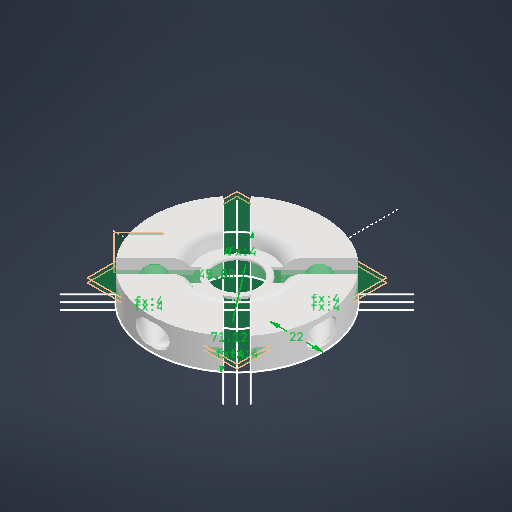
# Autodesk Inventor part: CENTER RING
Saved by Autodesk Inventor 2025 (Build 290162010, 162A)
## iProperties
Created: 2025-07-06
Part Number: CENTER RING
Material: Generic
Document SubType Name: Modeling
Designer: Jebediah Kerman
Density: 1 g/cm^3
Appearance: Default
Author: Jebediah Kerman
Autodesk Inventor part; units mm, degrees
ref_plane "YZ Plane" through (0, 0, 0) normal (1, 0, 0) x (0, 1, 0)
ref_plane "XZ Plane" through (0, 0, 0) normal (0, 1, 0) x (-1, 0, 0)
ref_plane "XY Plane" through (0, 0, 0) normal (0, 0, 1) x (1, 0, 0)
sketch "Sketch1" plane through (0, 0, 0) normal (0, 1, 0) x (-1, 0, 0)
  circle A0 centre (0, 0) radius 35.56
  circle A1 centre (0, 0) radius 13.56
  line L0 (0, 0) -> (36.4898, -36.4898)
  line L1 (0, 0) -> (51.6043, 0) construction
  line L2 (0, 0) -> (0, -67.3303) construction
  line L3 (0, 0) -> (-36.4898, -36.4898)
  line L4 (0, 0) -> (36.4898, 36.4898)
  line L5 (0, 0) -> (-36.4898, 36.4898)
  line L6 (-2.8284, 2.8284) -> (-39.3182, -33.6614)
  line L7 (2.8284, -2.8284) -> (-33.6614, -39.3182)
  line L8 (-2.8284, -2.8284) -> (-39.3182, 33.6614)
  line L9 (2.8284, 2.8284) -> (-33.6614, 39.3182)
  line L10 (2.8284, -2.8284) -> (39.3182, 33.6614)
  line L11 (-2.8284, 2.8284) -> (33.6614, 39.3182)
  line L12 (2.8284, 2.8284) -> (39.3182, -33.6614)
  line L13 (-2.8284, -2.8284) -> (33.6614, -39.3182)
  point P0 (11.9901, 6.3333)
  point P1 (27.8136, 22.1567)
  point P2 (22.1567, 27.8136)
  point P3 (6.3333, 11.9901)
  point P4 (6.3333, -11.9901)
  point P5 (22.1567, -27.8136)
  point P6 (27.8136, -22.1567)
  point P7 (11.9901, -6.3333)
  point P8 (-11.9901, -6.3333)
  point P9 (-27.8136, -22.1567)
  point P10 (-22.1567, -27.8136)
  point P11 (-6.3333, -11.9901)
  point P12 (-27.8136, 22.1567)
  point P13 (-11.9901, 6.3333)
  point P14 (-6.3333, 11.9901)
  point P15 (-22.1567, 27.8136)
  dimension "d0" = 71.12
  dimension "d1" = 22
  dimension "d4" = 45
  dimension "d5" = 4
  dimension "d6" = 4
  dimension "d7" = 4
  dimension "d8" = 4
  dimension "d9" = 4
  dimension "d10" = 4
  dimension "d11" = 4
  dimension "d12" = 4
  constraints: 28 end point, 8 parallel, 3 symmetric about line, 2 centre point, 1 coincident, 1 equal length, 1 horizontal, 1 vertical
  measures "d0" diameter of A0
  measures "d1" radial gap between concentric circles of A0 A1
  measures "d4" angle of L0 L1
  measures "d5" distance between parallel lines of L3 L6
  measures "d6" distance between parallel lines of L3 L7
  measures "d7" distance between parallel lines of L5 L8
  measures "d8" distance between parallel lines of L5 L9
  measures "d9" distance between parallel lines of L4 L10
  measures "d10" distance between parallel lines of L4 L11
  measures "d11" distance between parallel lines of L0 L12
  measures "d12" distance between parallel lines of L0 L13
extrude "Extrusion1" add sketch "Sketch1" along normal blind 13 contours A0 L12 A1 L10 | L10 A1 L4 A0 | A0 L0 A1 L12 | L4 A1 L11 A0 | A0 L13 A1 L0 | L11 A1 L9 A0 | A0 L7 A1 L13 | L9 A1 L5 A0 | A0 L3 A1 L7 | L5 A1 L8 A0 | A0 L6 A1 L3 | L8 A1 L6 A0
extrude "Extrusion2" cut sketch "Sketch1" along normal blind 13 contours L10 A1 L4 A0 | A0 L0 A1 L12 | L4 A1 L11 A0 | A0 L13 A1 L0 | L9 A1 L5 A0 | A0 L3 A1 L7 | L5 A1 L8 A0 | A0 L6 A1 L3
ref_plane "Work Plane1" through (-36.2988, 0, 13.6714) normal (-0.7071068, 0, -0.7071068) x (-0.7071068, 0, 0.7071068)
sketch "Sketch2" plane through (-36.2988, 0, 13.6714) normal (-0.7071068, 0, -0.7071068) x (-0.7071068, 0, 0.7071068)
  line L0 (0, 0) -> (-31.3343, 0) projected
  line L1 (-22.3777, 13) -> (-22.3777, 0) projected
  line L2 (0, 0) -> (-22.3777, 13) construction
  line L3 (0, 0) -> (0, 13) projected
  line L4 (-22.3777, 0) -> (0, 13) construction
  circle A0 centre (-11.1889, 6.5) radius 4.5
  point P0 (-35.3343, 0)
  dimension "d16" = 9
  constraints: 4 end point, 1 centre point, 1 coincident, 1 midpoint
  measures "d16" diameter of A0
extrude "Extrusion3" cut sketch "Sketch2" along normal blind 13 and the other way blind 50
mirror "Mirror1" about plane through (0, 0, 0) normal (1, 0, 0) of "Extrusion3"
mirror "Mirror2" about plane through (0, 0, 0) normal (0, 0, 1) of "Extrusion3", "Mirror1"
fillet "Fillet1" radius 6 4 edges at (13.56, 13, 0) (0, 13, 13.56) (-13.56, 13, 0) (0, 13, -13.56)
ref_plane "Work Plane3" through (0, 8.75, 0) normal (0, -1, 0) x (1, 0, 0)
ref_plane "Work Plane2" through (0, 7, 0) normal (0, -1, 0) x (1, 0, 0)
sketch "Sketch4" plane through (0, 8.75, 0) normal (0, -1, 0) x (1, 0, 0)
  circle A0 centre (0, 0) radius 11
  line L0 (27.8136, 22.1567) -> (11.9901, 6.3333) projected
  circle A1 centre (0, 0) radius 14.2522
  line L1 (11.9901, -6.3333) -> (27.8136, -22.1567) projected
  line L2 (12.5012, -6.8444) -> (-6.8444, 12.5012)
  line L3 (-12.5012, 6.8444) -> (6.8444, -12.5012)
  line L4 (-6.8444, -12.5012) -> (12.5012, 6.8444)
  line L5 (6.8468, 12.4999) -> (-12.4999, -6.8468)
  circle A2 centre (0, 0) radius 8.5
  point P0 (6.9302, -12.4538)
  point P1 (-12.4538, 6.9302)
  point P2 (-6.9302, 12.4538)
  point P3 (12.4538, 6.9302)
  point P4 (10.0741, -4.4173)
  point P5 (10.0741, 4.4173)
  point P6 (4.4199, 10.073)
  point P7 (-4.4173, 10.0741)
  point P8 (-10.0741, 4.4173)
  point P9 (-10.073, -4.4199)
  point P10 (-4.4173, -10.0741)
  point P11 (4.4173, -10.0741)
  point P12 (5.6569, 0)
  point P13 (0, -5.6569)
  point P14 (-5.655, -0.0019)
  point P15 (0.0019, 5.655)
  dimension "d28" = 22
  dimension "d33" = 17
  constraints: 8 end point, 3 coincident, 3 point on line, 2 centre point, 2 parallel, 1 collinear, 14 other
  measures "d28" diameter of A0
  measures "d33" diameter of A2
extrude "Extrusion5" add sketch "Sketch4" against normal blind 1 contours A0 L2 A2 L4 | A0 L4 L0 A1 L1 L2 | L4 A2 L5 A0 | A0 L3 A2 L2 | L5 A2 L2 A0 | A0 L2 A1 L5 | L3 A1 L4 A0 | A0 L4 A2 L3 | L2 A2 L3 A0 | A0 L5 A2 L4 | L3 A2 L5 A0 | A0 L5 A1 L3
fillet "Fillet3" radius 0.5 1 edges at (7.7782, 9.75, -7.7782)
fillet "Fillet4" radius 0.5 2 edges at (-8.5, 8.75, 0) (-8.5, 9.75, 0)
equation "\"d5\" = d11"
equation "\"d6\" = d11"
equation "\"d7\" = d11"
equation "\"d8\" = d12"
equation "\"d9\" = d12"
equation "\"d10\" = d11"
equation "\"d12\" = d11"
body "Solid1"
